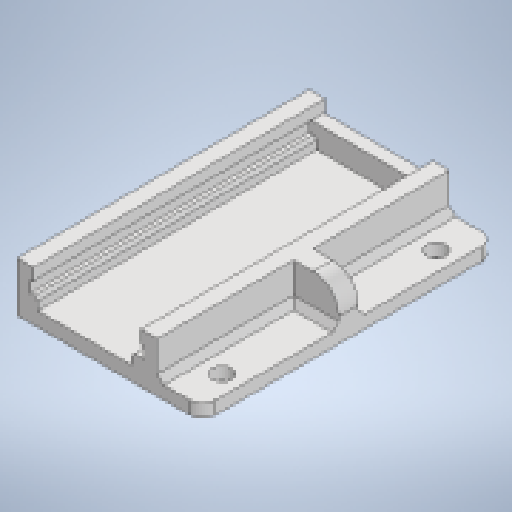
# Autodesk Inventor part: relay_case
Saved by Autodesk Inventor 2025.1 (Build 291241000, 241)
## iProperties
Created: 2026-05-31
Part Number: relay_case
Material: Generic
Document SubType Name: Modeling
Designer: User
Density: 1 g/cm^3
Appearance: Default
Author: User
Autodesk Inventor part; units mm, degrees
ref_plane "YZ Plane" through (0, 0, 0) normal (1, 0, 0) x (0, 1, 0)
ref_plane "XZ Plane" through (0, 0, 0) normal (0, 1, 0) x (-1, 0, 0)
ref_plane "XY Plane" through (0, 0, 0) normal (0, 0, 1) x (1, 0, 0)
sketch "Sketch1" plane through (0, 0, 0) normal (0, 0, 1) x (1, 0, 0)
  line L0 (0, 0) -> (0, 1.3) projected
  line L1 (0, 0) -> (17.2, 0) projected
  line L2 (17.2, 0) -> (17.2, 1.3) projected
  line L3 (0, 1.3) -> (17.2, 1.3) projected
  line L4 (-0.2, -0.2) -> (-0.2, 1.5)
  line L5 (17.4, 1.5) -> (17.4, -0.2)
  line L6 (-2.2, 3.5) -> (-2.2, -2.2)
  line L7 (19.4, -2.2) -> (19.4, 3.5)
  line L8 (0.49, 2.4) -> (0.49, 1.65)
  line L9 (0.29, 2.4) -> (0.29, 1.65)
  line L10 (16.69, 2.4) -> (16.69, 1.65)
  line L11 (16.89, 2.4) -> (16.89, 1.65)
  line L12 (16.89, 1.5) -> (16.89, 3.5)
  line L13 (0.29, 1.5) -> (0.29, 3.5)
  line L14 (19.4, 3.5) -> (16.89, 3.5)
  line L15 (0.29, 3.5) -> (-2.2, 3.5)
  line L16 (-0.2, 1.5) -> (0.29, 1.5)
  line L17 (16.89, 1.5) -> (17.4, 1.5)
  line L18 (15.45, -2) -> (0.93, -2)
  line L19 (-2, -2) -> (-2, 3.3)
  line L20 (19.2, 3.3) -> (19.2, -2)
  line L21 (1.13, -0.1) -> (1.13, 0)
  line L22 (0.93, -0.1) -> (0.93, 0)
  line L23 (0.93, 0) -> (0.93, -2)
  line L24 (15.25, -0.1) -> (15.25, 1.4)
  line L25 (15.45, -0.1) -> (15.45, 1.4)
  line L26 (15.45, 1.3) -> (15.45, -2)
  line L27 (-2.2, -2.2) -> (-2.2, -4.2)
  line L28 (-2.2, -4.2) -> (19.4, -4.2)
  line L29 (19.4, -4.2) -> (19.4, -2.2)
  line L30 (17.4, -0.2) -> (15.45, -0.2)
  line L31 (0.93, -0.2) -> (-0.2, -0.2)
  line L32 (0.49, -2.2) -> (1.13, -2.2)
  line L33 (15.25, -2.2) -> (16.89, -2.2)
  line L34 (-2.2, -2.2) -> (-2, -2.2)
  line L35 (-0.2, -2.2) -> (0.29, -2.2)
  line L36 (17.2, -2.2) -> (17.4, -2.2)
  line L37 (19.2, -2.2) -> (19.4, -2.2)
  line L38 (0.29, 3.3) -> (1.13, 3.3)
  line L39 (15.25, 3.3) -> (16.89, 3.3)
  dimension "d2" = 0.2
  dimension "d3" = 0.2
  dimension "d4" = 2
  dimension "d5" = 0.2
  dimension "d6" = 0.2
  dimension "d7" = 2
  constraints: 72 end point, 20 point on line, 5 perpendicular, 5 vertical, 4 parallel, 8 other
  measures "d2" distance between parallel lines of L8 L9
  measures "d3" distance between parallel lines of L10 L11
  measures "d4" distance between parallel lines of L1 L18
  measures "d5" distance between parallel lines of L21 L22
  measures "d6" distance between parallel lines of L24 L25
  measures "d7" distance of L6.end L27.end
ref_plane "Work Plane1" through (0, 0, -43.05) normal (0, 0, -1) x (0, 1, 0)
extrude "Extrusion1" add sketch "Sketch1" against normal up to surface (43.05 mm away) contours L23 L18 L26 L30 L5 L17 L12 L11 L14 L7 L29 L28 L27 L6 L15 L13 L9 L16 L4 L31
chamfer "Chamfer1" distance 0.5 angle 45 2 edges at (15.45, -0.2, -21.525) (0.93, -0.2, -21.525)
chamfer "Chamfer2" distance 0.2 angle 45 2 edges at (0.29, 1.5, -21.525) (16.89, 1.5, -21.525)
sketch "Sketch2" plane through (19.4, -4.2, -43.05) normal (0, 0, -1) x (-1, 0, 0)
  line L0 (2.51, 5.9) -> (2.31, 5.7) projected
  line L1 (2.51, 7.7) -> (2.51, 5.9) projected
  line L2 (0, 7.7) -> (2.51, 7.7) projected
  line L3 (0, 0) -> (0, 7.7) projected
  line L4 (21.6, 0) -> (0, 0) projected
  line L5 (21.6, 7.7) -> (21.6, 0) projected
  line L6 (19.11, 7.7) -> (21.6, 7.7) projected
  line L7 (19.11, 5.9) -> (19.11, 7.7) projected
  line L8 (19.31, 5.7) -> (19.11, 5.9) projected
  line L9 (19.6, 5.7) -> (19.31, 5.7) projected
  line L10 (19.6, 4) -> (19.6, 5.7) projected
  line L11 (18.97, 4) -> (19.6, 4) projected
  line L12 (18.47, 3.5) -> (18.97, 4) projected
  line L13 (18.47, 2.2) -> (18.47, 3.5) projected
  line L14 (3.95, 2.2) -> (18.47, 2.2) projected
  line L15 (3.95, 3.5) -> (3.95, 2.2) projected
  line L16 (3.45, 4) -> (3.95, 3.5) projected
  line L17 (2, 4) -> (3.45, 4) projected
  line L18 (2, 5.7) -> (2, 4) projected
  line L19 (2.31, 5.7) -> (2, 5.7) projected
  line L20 (0, 5.7) -> (21.6, 5.7)
  point P0 (19.4, 4.2)
  constraints: 2 end point, 2 point on line, 1 perpendicular
extrude "Extrusion2" add sketch "Sketch2" along normal blind 2
sketch "Sketch3" plane through (-2.2, -4.2, 0) normal (0, -1, 0) x (1, 0, 0)
  line L0 (21.6, 0) -> (21.6, -45.05) projected
  line L1 (21.6, 0) -> (26.6, 0)
  line L2 (28.6, -2) -> (28.6, -43.05)
  line L3 (26.6, -45.05) -> (21.6, -45.05)
  line L4 (28.6, 0) -> (25.6, 0)
  line L5 (25.6, 0) -> (25.6, -45.05)
  line L6 (25.6, 0) -> (25.6, -6)
  line L7 (25.6, -45.05) -> (25.6, -39.05)
  circle A0 centre (25.6, -6) radius 1.5
  circle A1 centre (25.6, -39.05) radius 1.5
  arc A2 (28.6, -2) -> (26.6, 0) centre (26.6, -2) ccw
  arc A3 (26.6, -45.05) -> (28.6, -43.05) centre (26.6, -43.05) ccw
  point P0 (2.2, 0)
  dimension "d18" = 7
  dimension "d19" = 3
  dimension "d20" = 6
  dimension "d21" = 6
  dimension "d22" = 3
  dimension "d23" = 3
  dimension "d24" = 2
  constraints: 14 end point, 6 point on line, 4 centre point, 4 point on circle, 4 tangent, 3 perpendicular, 2 coincident, 1 equal radius, 1 horizontal
  measures "d18" distance of L0.start L4.start
  measures "d19" distance of L4.start L4.end
  measures "d20" distance of L4.end L6.end
  measures "d21" distance of L5.end L7.end
  measures "d22" diameter of A0
  measures "d23" diameter of A1
  measures "d24" radius of A2
extrude "Extrusion3" add sketch "Sketch3" against normal blind 2 contours L1 L5 A0 A1 L3 L0 | L1 A2 L2 A3 L3 L5 A1 A0
chamfer "Chamfer3" distance 1 angle 45 1 edges at (19.4, -2.2, -22.525)
sketch "Sketch4" plane through (26.4, -4.2, -2) normal (1, 0, 0) x (0, 0, -1)
  line L0 (0, 2) -> (41.05, 2) projected
  line L1 (20.525, 2) -> (20.525, 7.7)
  line L2 (-2, 7.7) -> (43.05, 7.7) projected
  line L3 (22.025, 7.7) -> (19.025, 7.7)
  line L4 (19.025, 7.7) -> (19.025, 2)
  line L5 (19.025, 2) -> (22.025, 2)
  line L6 (22.025, 2) -> (22.025, 7.7)
  line L7 (22.025, 7.7) -> (19.025, 2) construction
  line L8 (19.025, 7.7) -> (22.025, 2) construction
  point P0 (-2, 4.2)
  point P1 (20.525, 4.85)
  point P2 (19.025, 7.7)
  point P3 (22.025, 2)
  point P4 (22.025, 7.7)
  dimension "d30" = 3
  constraints: 14 end point, 5 midpoint, 2 parallel, 1 horizontal, 1 perpendicular, 1 point on line
  measures "d30" distance of L5.end L4.end
extrude "Extrusion4" add sketch "Sketch4" against normal up to surface (7 mm away)
fillet "Fillet1" radius 4 1 edges at (26.4, 3.5, -22.525)
chamfer "Chamfer4" distance 1 angle 45 2 edges at (23.4, -2.2, -21.025) (23.4, -2.2, -24.025)
body "Solid1"
